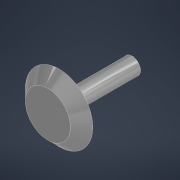
# Autodesk Inventor part: P006
Saved by Autodesk Inventor 2021.3 (Build 253353000, 353)
## iProperties
Company: HES-SO
Created: 2022-03-24
Part Number: P006
Material: Aluminium
Document SubType Name: Modeling
Designer: HER & ZAE
Density: 2.7 g/cm^3
Appearance: Aluminum - Dark
Mass: 0.677877 g
Surface Area: 3.74743 cm^2
Volume: 0.251066 cm^3
Author: HER & ZAE
Title: Soupape IN
Autodesk Inventor part; units mm, degrees
ref_plane "YZ Plane" through (0, 0, 0) normal (1, 0, 0) x (0, 1, 0)
ref_plane "XZ Plane" through (0, 0, 0) normal (0, 1, 0) x (-1, 0, 0)
ref_plane "XY Plane" through (0, 0, 0) normal (0, 0, 1) x (1, 0, 0)
sketch "Sketch2" plane through (0, 0, 0) normal (0, 0, 1) x (1, 0, 0)
  line L0 (0, -3.6) -> (0, 21.6) construction
  line L1 (-7.2, 0) -> (1.2, 0) construction
  line L2 (0, 0) -> (-6, 0)
  line L3 (-6, 2) -> (-1.5, 2)
  line L4 (-1.5, 2) -> (-1.5, 4.114)
  line L5 (-1.5, 4.7135) -> (-1.5, 15)
  line L6 (-1.5, 15) -> (0, 15)
  line L7 (0, 0) -> (-6, 0)
  line L8 (-6, 2) -> (-6, 0)
  line L9 (-1.5, 3.3248) -> (-1.5, 5.5716)
  line L10 (0, 15) -> (0, 0)
  point P0 (-1.5, 4.114)
  dimension "d0" = 1.5
  dimension "d1" = 6
  dimension "d3" = 2
  dimension "HighRod" = 13
  constraints: 18 end point, 6 point on line, 4 perpendicular, 1 horizontal, 1 parallel
  measures "d0" distance between parallel lines of L5 L0
  measures "d1" distance between parallel lines of L8 L0
  measures "d3" distance between parallel lines of L1 L3
  measures "HighRod" distance between parallel lines of L3 L6
revolve "Revolution1" add sketch "Sketch2" angle 360 about axis through (0, -10, 0) along (0, 1, 0)
chamfer "Chamfer_top" [suppressed]
chamfer "Chamfer_bottom" distance 2 angle 45 1 edges at (6, 0, 0)
body "Solid1"
